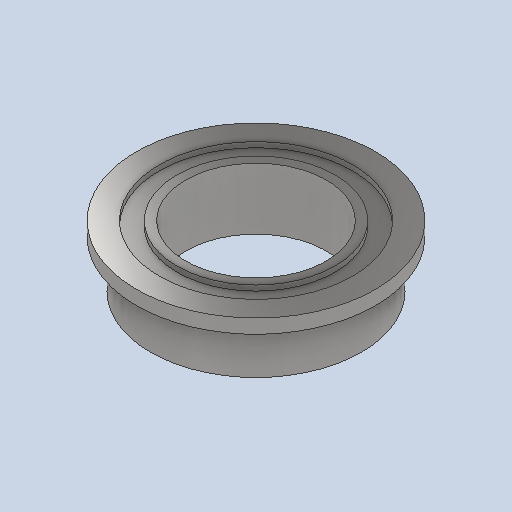
# Autodesk Inventor part: Bearing_MF128ZZ
Saved by Autodesk Inventor 2022 (Build 260153000, 153)
## iProperties
Created: 2020-11-19
Part Number: Bearing_MF128ZZ
Material: ステンレス鋼
Document SubType Name: Modeling
Designer: yuta2
Mass: 1.15 g
Surface Area: 4.13936 cm^2
Volume: 0.245647 cm^3
Density: 4.68151 g/cm^3
Appearance: 半つや出し
Author: yuta2
Autodesk Inventor part; units mm, degrees
ref_plane "YZ Plane" through (0, 0, 0) normal (1, 0, 0) x (0, 1, 0)
ref_plane "XZ Plane" through (0, 0, 0) normal (0, 1, 0) x (-1, 0, 0)
ref_plane "XY Plane" through (0, 0, 0) normal (0, 0, 1) x (1, 0, 0)
sketch "スケッチ1" plane through (0, 0, 0) normal (0, 1, 0) x (-1, 0, 0)
  circle A0 centre (0, 0) radius 4
  circle A1 centre (0, 0) radius 6
  dimension "d0" = 8
  dimension "d1" = 12
  constraints: 2 centre point, 2 coincident
  measures "d0" diameter of A0
  measures "d1" diameter of A1
extrude "押し出し1" add sketch "スケッチ1" along normal blind 3.5
sketch "スケッチ2" plane through (0, 3.5, 0) normal (0, 1, 0) x (1, 0, 0)
  circle A0 centre (0, 0) radius 6
  circle A1 centre (0, 0) radius 6.8
  circle A2 centre (0, 0) radius 6 projected
  dimension "d4" = 13.6
  constraints: 2 centre point, 2 coincident, 1 concentric
  measures "d4" diameter of A1
extrude "押し出し2" add sketch "スケッチ2" against normal blind 0.8
sketch "スケッチ3" plane through (0, 3.5, 0) normal (0, 1, 0) x (1, 0, 0)
  circle A0 centre (0, 0) radius 4 projected
  circle A1 centre (0, 0) radius 4.5
  circle A2 centre (0, 0) radius 5.5
  dimension "d7" = 9
  dimension "d8" = 11
  constraints: 2 centre point, 2 coincident
  measures "d7" diameter of A1
  measures "d8" diameter of A2
extrude "押し出し3" cut sketch "スケッチ3" against normal blind 0.3 contours A2
sketch "スケッチ4" plane through (0, 0, 0) normal (0, -1, 0) x (1, 0, 0)
  circle A0 centre (0, 0) radius 4 projected
  circle A1 centre (0, 0) radius 4.5
  circle A2 centre (0, 0) radius 5.5
  dimension "d11" = 9
  dimension "d12" = 11
  constraints: 2 centre point, 2 coincident
  measures "d11" diameter of A1
  measures "d12" diameter of A2
extrude "押し出し4" cut sketch "スケッチ4" against normal blind 0.3 contours A2
